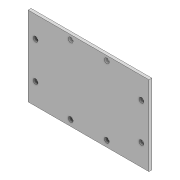
# Autodesk Inventor part: PlacaReductor
Saved by Autodesk Inventor 2021 (Build 250183000, 183)
## iProperties
Created: 2021-08-21
Part Number: PlacaReductor
Material: Generic
Document SubType Name: Sheet Metal
Designer: Santiago Suárez
Density: 1 g/cm^3
Sheet Metal Rule: Default_mm
Appearance: Default
Author: Santiago Suárez
Autodesk Inventor part; units mm, degrees
ref_plane "YZ Plane" through (0, 0, 0) normal (1, 0, 0) x (0, 1, 0)
ref_plane "XZ Plane" through (0, 0, 0) normal (0, 1, 0) x (-1, 0, 0)
ref_plane "XY Plane" through (0, 0, 0) normal (0, 0, 1) x (1, 0, 0)
sketch "Sketch1" plane through (0, 0, 0) normal (0, 0, 1) x (1, 0, 0)
  line L0 (-197.5, 130) -> (197.5, 130)
  line L1 (197.5, 130) -> (197.5, -130)
  line L2 (197.5, -130) -> (-197.5, -130)
  line L3 (-197.5, -130) -> (-197.5, 130)
  point P0 (0, 0)
  dimension "d0" = 395
  dimension "d1" = 260
  dimension "d2" = 130
  dimension "d3" = 197.5
  measures "d0" distance of L0.start L0.end
  measures "d1" distance of L2.end L0.start
  measures "d2" distance from line of point (0, 0) L0
  measures "d3" distance from line of point (0, 0) L3
extrude "Plate1" add sketch "Sketch1" along normal blind 9.5
sketch "Sketch2" plane through (0, 0, 9.5) normal (0, 0, 1) x (1, 0, 0)
  line L0 (-58.2, 115) -> (59.8, 115)
  line L1 (59.8, 115) -> (59.8, -110)
  line L2 (59.8, -110) -> (-58.2, -110)
  line L3 (-58.2, -110) -> (-58.2, 115)
  line L4 (-197.5, -130) -> (-197.5, 130) projected
  line L5 (197.5, -130) -> (-197.5, -130) projected
  line L6 (-173, 60) -> (173, 60)
  line L7 (173, 60) -> (173, -60)
  line L8 (173, -60) -> (-173, -60)
  line L9 (-173, -60) -> (-173, 60)
  line L10 (197.5, 130) -> (197.5, -130) projected
  point P0 (0, 0)
  dimension "d5" = 118
  dimension "d6" = 139.3
  dimension "d7" = 225
  dimension "d8" = 20
  dimension "d16" = 24.5
  dimension "d17" = 120
  dimension "d18" = 60
  dimension "d19" = 24.5
  constraints: 16 end point, 8 coincident, 4 parallel, 2 horizontal, 2 perpendicular
  measures "d5" distance of L1.end L2.end
  measures "d6" distance between parallel lines of L4 L3
  measures "d7" distance of L2.end L0.start
  measures "d8" distance between parallel lines of L5 L2
  measures "d16" distance between parallel lines of L4 L9
  measures "d17" distance of L8.end L6.start
  measures "d18" distance from line of point (0, 0) L6
  measures "d19" distance between parallel lines of L10 L7
hole "Hole1" at (-58.2, -110, 9.5) at (-58.2, 115, 9.5) at (59.8, 115, 9.5) at (59.8, -110, 9.5) at (-173, 60, 9.5) at (-173, -60, 9.5) at (173, 60, 9.5) at (173, -60, 9.5) direction (0, 0, -1) diameter 16 depth 9.5
equation "\"d18\" = 0.5 * d17"
equation "\"d14\" = Thickness"
equation "\"d4\" = Thickness"
equation "\"d2\" = 0.5 * d1"
equation "\"d3\" = 0.5 * d0"
equation "\"BendRadius\" = Thickness"
equation "\"BendReliefWidth\" = Thickness"
equation "\"BendReliefDepth\" = 0.5 * Thickness"
equation "\"CornerReliefSize\" = 4 * Thickness"
equation "\"MinimumRemnant\" = 2 * Thickness"
equation "\"TransitionRadius\" = BendRadius"
equation "\"JacobiRadiusSize\" = BendRadius"
equation "\"GapSize\" = Thickness"
equation "\"Thickness\" = 9.5"
body "Solid1"
